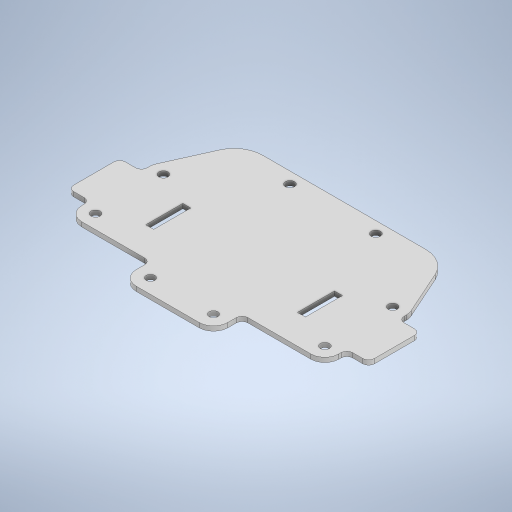
# Autodesk Inventor part: ty
Saved by Autodesk Inventor 2023 (Build 270158000, 158)
## iProperties
Created: 2024-03-30
Part Number: ty
Material: Ogólny
Document SubType Name: Modeling
Designer: Kamil
Density: 1 g/cm^3
Appearance: Domyślna
Author: Kamil
Autodesk Inventor part; units mm, degrees
ref_plane "YZ Plane" through (0, 0, 0) normal (1, 0, 0) x (0, 1, 0)
ref_plane "XZ Plane" through (0, 0, 0) normal (0, 1, 0) x (-1, 0, 0)
ref_plane "XY Plane" through (0, 0, 0) normal (0, 0, 1) x (1, 0, 0)
sketch "Szkic1" plane through (0, 0, 0) normal (0, 1, 0) x (-1, 0, 0)
  line L0 (52.5, 25) -> (-52.5, 25)
  line L1 (-52.5, 25) -> (-52.5, -25)
  line L2 (-52.5, -25) -> (52.5, -25)
  line L3 (52.5, -25) -> (52.5, 25)
  line L4 (52.5, 25) -> (-52.5, -25) construction
  line L5 (-52.5, 25) -> (52.5, -25) construction
  point P0 (0, 0)
  dimension "d0" = 105
  dimension "d1" = 50
  constraints: 12 end point, 2 midpoint, 2 parallel, 1 horizontal, 1 perpendicular
  measures "d0" distance of L1.end L2.end
  measures "d1" distance of L2.end L0.start
extrude "Wyciągnięcie proste1" add sketch "Szkic1" along normal blind 1.6
sketch "Szkic5" plane through (0, 1.6, 0) normal (0, 1, 0) x (1, 0, 0)
  circle A0 centre (-40.05, 11.85) radius 1.6 projected
  circle A1 centre (-40.05, -11.85) radius 1.6 projected
  circle A2 centre (40.05, 11.85) radius 1.6 projected
  circle A3 centre (40.05, -11.85) radius 1.6 projected
  point P0 (0, 0)
extrude "Wyciągnięcie proste4" cut sketch "Szkic5" against normal blind 10
sketch "Szkic6" plane through (0, 1.6, 0) normal (0, 1, 0) x (1, 0, 0)
  line L0 (52.5, 25) -> (-52.5, 25) projected
  line L1 (52.5, 25) -> (-52.5, 25)
  line L2 (-52.5, 25) -> (-52.5, 35)
  line L3 (-52.5, 35) -> (52.5, 35)
  line L4 (52.5, 35) -> (52.5, 25)
  point P0 (0, 0)
  point P1 (-52.5, 25)
  dimension "d15" = 10
  constraints: 8 end point, 2 parallel, 1 horizontal, 1 perpendicular
  measures "d15" distance of L1.end L2.end
extrude "Wyciągnięcie proste5" add sketch "Szkic6" against normal up to surface (1.6 mm away)
sketch "Szkic7" plane through (0, 1.6, 0) normal (0, 1, 0) x (1, 0, 0)
  arc A0 (35.2, -11.85) -> (44.9, -11.85) centre (40.05, -11.85) ccw projected
  arc A1 (46.9, -9) -> (44.9, -11) centre (46.9, -11) ccw projected
  line L0 (44.9, -11) -> (44.9, -11.85) projected
  line L1 (52.5, -9) -> (35.2, -9) projected
  line L2 (52.5, 9) -> (35.2, 9) projected
  arc A2 (44.9, 11) -> (46.9, 9) centre (46.9, 11) ccw projected
  arc A3 (44.9, 11.85) -> (35.2, 11.85) centre (40.05, 11.85) ccw projected
  line L3 (-52.5, -9) -> (-35.2, -9) projected
  arc A4 (-44.9, -11) -> (-46.9, -9) centre (-46.9, -11) ccw projected
  arc A5 (-44.9, -11.85) -> (-35.2, -11.85) centre (-40.05, -11.85) ccw projected
  line L4 (-52.5, 9) -> (-35.2, 9) projected
  arc A6 (-46.9, 9) -> (-44.9, 11) centre (-46.9, 11) ccw projected
  arc A7 (-35.2, 11.85) -> (-44.9, 11.85) centre (-40.05, 11.85) ccw projected
  line L5 (40.05, -16.7) -> (-40.05, -16.7)
  line L6 (52.5, 35) -> (-52.5, 35) projected
  circle A8 centre (11, -115) radius 1.55 projected
  circle A9 centre (-11, -115) radius 1.55 projected
  circle A10 centre (-11, -21.7) radius 1.55
  circle A11 centre (11, -21.7) radius 1.55
  circle A12 centre (-11, -21.7) radius 5
  circle A13 centre (11, -21.7) radius 5
  line L7 (16, -21.7) -> (16, -16.7)
  line L8 (-16, -21.7) -> (-16, -16.7)
  line L9 (11, -26.7) -> (-11, -26.7)
  circle A14 centre (40.05, 11.85) radius 1.6 projected
  circle A15 centre (-40.05, 11.85) radius 1.6 projected
  circle A16 centre (40.05, -11.85) radius 1.6 projected
  circle A17 centre (-40.05, -11.85) radius 1.6 projected
  line L10 (52.5, -25) -> (52.5, 35) projected
  line L11 (52.5, 35) -> (-52.5, 35) projected
  line L12 (-52.5, 35) -> (-52.5, -25) projected
  line L13 (-52.5, -25) -> (52.5, -25) projected
  arc A18 (-44.9, -11.85) -> (-35.2, -11.85) centre (-40.05, -11.85) ccw projected
  arc A19 (-44.9, -11.85) -> (-35.2, -11.85) centre (-40.05, -11.85) ccw projected
  line L14 (-44.9, -11.85) -> (-44.9, -11) projected
  point P0 (0, 0)
  point P1 (14.7563, -25)
  point P2 (-14.7563, -25)
  dimension "d18" = 3.1
  dimension "d19" = 3.1
  dimension "d20" = 10
  dimension "d21" = 10
  constraints: 8 end point, 6 point on circle, 4 centre point, 3 tangent, 2 coincident, 2 point on line, 2 vertical alignment, 1 perpendicular, 1 vertical
  measures "d18" diameter of A11
  measures "d19" diameter of A10
  measures "d20" diameter of A12
  measures "d21" diameter of A13
extrude "Wyciągnięcie proste6" cut sketch "Szkic7" against normal blind 10 contours A0 L0 A1 L1 L10 L13 A13 L7 L5 | L8 A12 L13 L12 L3 A4 L14 A5 L5 | A10 | A11
sketch "Szkic8" plane through (0, 1.6, 0) normal (0, 1, 0) x (1, 0, 0)
  circle A0 centre (11, -21.7) radius 1.55 projected
  circle A1 centre (-11, -21.7) radius 1.55 projected
  arc A2 (14.7563, -25) -> (16, -21.7) centre (11, -21.7) ccw projected
  circle A3 centre (11, -21.7) radius 5
  line L0 (-14.7563, -25) -> (14.7563, -25) projected
  circle A4 centre (-11, -21.7) radius 5
  line L1 (11, -26.7) -> (-11, -26.7)
  point P0 (0, 0)
  constraints: 4 point on circle, 2 centre point, 2 coincident, 2 end point, 1 tangent
extrude "Wyciągnięcie proste7" add sketch "Szkic8" against normal up to surface (1.6 mm away) contours A3 L0 | L1 A4 L0 A3 | A4 L0 picked at (-10.008, -25.2393)
sketch "Szkic9" plane through (0, 1.6, 0) normal (0, 1, 0) x (1, 0, 0)
  circle A0 centre (11, -21.7) radius 1.5 projected
  circle A1 centre (-11, -21.7) radius 1.5 projected
  circle A2 centre (-15, 31) radius 1.6
  circle A3 centre (15, 31) radius 1.6
  line L0 (15, 31) -> (-15, 31)
  line L1 (52.5, 35) -> (-52.5, 35) projected
  point P0 (0, 0)
  point P1 (0, 35)
  point P2 (0, 31)
  dimension "d26" = 3.2
  dimension "d27" = 3.2
  dimension "d28" = 30
  dimension "d29" = 4
  constraints: 2 centre point, 2 end point, 2 midpoint, 1 horizontal, 1 horizontal alignment, 1 vertical alignment
  measures "d26" diameter of A2
  measures "d27" diameter of A3
  measures "d28" distance of L0.end L0.start
  measures "d29" distance between parallel lines of L1 L0
extrude "Wyciągnięcie proste8" cut sketch "Szkic9" against normal through all contours A2 | A3
sketch "Szkic10" plane through (0, 1.6, 0) normal (0, 1, 0) x (1, 0, 0)
  line L0 (-27.4, 5.9859) -> (-27.4, -5.9859) projected
  line L1 (-25.6, 5.9859) -> (-27.4, 5.9859) projected
  line L2 (-25.6, -5.9859) -> (-25.6, 5.9859) projected
  line L3 (-27.4, -5.9859) -> (-25.6, -5.9859) projected
  line L4 (27.4, -5.9859) -> (27.4, 5.9859) projected
  line L5 (25.6, -5.9859) -> (27.4, -5.9859) projected
  line L6 (25.6, 5.9859) -> (25.6, -5.9859) projected
  line L7 (27.4, 5.9859) -> (25.6, 5.9859) projected
  line L8 (-27.9, -6.4859) -> (-27.9, 6.4859)
  line L9 (-27.9, 6.4859) -> (-25.1, 6.4859)
  line L10 (-25.1, 6.4859) -> (-25.1, -6.4859)
  line L11 (-25.1, -6.4859) -> (-27.9, -6.4859)
  line L12 (25.1, -6.4859) -> (27.9, -6.4859)
  line L13 (27.9, -6.4859) -> (27.9, 6.4859)
  line L14 (27.9, 6.4859) -> (25.1, 6.4859)
  line L15 (25.1, 6.4859) -> (25.1, -6.4859)
  point P0 (0, 0)
  dimension "d32" = 0.5
  dimension "d33" = 0.5
  constraints: 16 end point, 6 other
  measures "d32" distance between parallel lines of L0 L8
  measures "d33" distance between parallel lines of L6 L15
extrude "Wyciągnięcie proste9" cut sketch "Szkic10" against normal blind 10 contours L1 L2 L3 L0 | L5 L6 L7 L4 | L8 L9 L10 L11 | L15 L14 L13 L12
sketch "Szkic11" plane through (0, 1.6, 0) normal (0, 1, 0) x (1, 0, 0)
  circle A0 centre (40.05, 11.85) radius 1.6 projected
  line L0 (52.5, 9) -> (46.9, 9) projected
  line L1 (52.5, 9) -> (52.5, 6) projected
  line L2 (52.5, 6) -> (35.2, 6) projected
  line L3 (35.2, 11.85) -> (35.2, 6) projected
  arc A1 (44.9, 11.85) -> (35.2, 11.85) centre (40.05, 11.85) ccw projected
  line L4 (44.9, 11.85) -> (44.9, 11) projected
  arc A2 (44.9, 11) -> (46.9, 9) centre (46.9, 11) ccw projected
  circle A3 centre (-40.05, 11.85) radius 1.6 projected
  line L5 (-35.2, 6) -> (-35.2, 11.85) projected
  line L6 (-52.5, 6) -> (-35.2, 6) projected
  line L7 (-52.5, 9) -> (-52.5, 6) projected
  line L8 (-52.5, 9) -> (-46.9, 9) projected
  arc A4 (-46.9, 9) -> (-44.9, 11) centre (-46.9, 11) ccw projected
  line L9 (-44.9, 11.85) -> (-44.9, 11) projected
  arc A5 (-35.2, 11.85) -> (-44.9, 11.85) centre (-40.05, 11.85) ccw projected
  line L10 (44.4767, 13.8317) -> (35, 35)
  line L11 (-52.5, 35) -> (52.5, 35) projected
  circle A6 centre (15, 31) radius 1.6 projected
  line L12 (-45.0282, 12.5998) -> (-35, 35)
  circle A7 centre (-15, 31) radius 1.6 projected
  line L13 (-27.9, 6.4859) -> (-25.1, 6.4859) projected
  line L14 (-25.1, 6.4859) -> (-25.1, -6.4859) projected
  line L15 (-25.1, -6.4859) -> (-27.9, -6.4859) projected
  line L16 (-27.9, -6.4859) -> (-27.9, 6.4859) projected
  line L17 (25.1, 6.4859) -> (27.9, 6.4859) projected
  line L18 (27.9, 6.4859) -> (27.9, -6.4859) projected
  line L19 (27.9, -6.4859) -> (25.1, -6.4859) projected
  line L20 (25.1, -6.4859) -> (25.1, 6.4859) projected
  circle A8 centre (15, 31) radius 1.6 projected
  circle A9 centre (-15, 31) radius 1.6 projected
  line L21 (46.9, -9) -> (52.5, -9) projected
  line L22 (52.5, -9) -> (52.5, 35) projected
  line L23 (52.5, 35) -> (-52.5, 35) projected
  line L24 (-52.5, 35) -> (-52.5, -9) projected
  line L25 (-52.5, -9) -> (-46.9, -9) projected
  arc A10 (-44.9, -11) -> (-46.9, -9) centre (-46.9, -11) ccw projected
  line L26 (-44.9, -11) -> (-44.9, -11.85) projected
  arc A11 (-44.9, -11.85) -> (-40.05, -16.7) centre (-40.05, -11.85) ccw projected
  line L27 (-40.05, -16.7) -> (-16, -16.7) projected
  line L28 (-16, -16.7) -> (-16, -21.7) projected
  arc A12 (-16, -21.7) -> (-11, -26.7) centre (-11, -21.7) ccw projected
  line L29 (-11, -26.7) -> (11, -26.7) projected
  arc A13 (11, -26.7) -> (16, -21.7) centre (11, -21.7) ccw projected
  line L30 (16, -21.7) -> (16, -16.7) projected
  line L31 (16, -16.7) -> (40.05, -16.7) projected
  arc A14 (40.05, -16.7) -> (44.9, -11.85) centre (40.05, -11.85) ccw projected
  line L32 (44.9, -11.85) -> (44.9, -11) projected
  arc A15 (46.9, -9) -> (44.9, -11) centre (46.9, -11) ccw projected
  circle A16 centre (11, -21.7) radius 1.55 projected
  circle A17 centre (-11, -21.7) radius 1.55 projected
  circle A18 centre (40.05, 11.85) radius 1.6 projected
  circle A19 centre (-40.05, 11.85) radius 1.6 projected
  circle A20 centre (40.05, -11.85) radius 1.6 projected
  circle A21 centre (-40.05, -11.85) radius 1.6 projected
  point P0 (0, 0)
  point P1 (-44.4767, 13.8317)
  point P2 (52.5, 35)
  dimension "d36" = 20
  dimension "d37" = 20
  constraints: 4 end point, 2 point on line, 2 tangent, 1 point on circle
  measures "d36" horizontal distance of L10.end A6.centre
  measures "d37" horizontal distance of L12.end A7.centre
extrude "Wyciągnięcie proste10" cut sketch "Szkic11" against normal blind 10 contours L0 A2 L4 A1 L10 L11 L22 | L12 A5 L9 A4 L8 L24 L11
fillet "Zaokrąglenie2" radius 10 2 edges at (35, 0.8, -35) (-35, 0.8, -35)
fillet "Zaokrąglenie3" radius 2 6 edges at (52.5, 0.8, 9) (52.5, 0.8, -9) (-52.5, 0.8, 9) (-52.5, 0.8, -9) (16, 0.8, 16.7) (-16, 0.8, 16.7)
